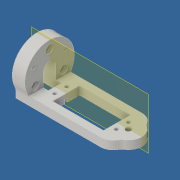
# Autodesk Inventor part: ServoMount
Saved by Autodesk Inventor 2016 SP1 (Build 200210100, 210)
## iProperties
Created: 2016-03-20
Part Number: ServoMount
Material: ABS-Kunststoff
Document SubType Name: Modeling
Designer: 4ndreas
Density: 1.06 g/cm^3
Appearance: Glatt - weiß
Mass: 21.5528 g
Surface Area: 97.0469 cm^2
Volume: 20.3328 cm^3
Author: 4ndreas
Autodesk Inventor part; units mm, degrees
ref_plane "YZ Plane" through (0, 0, 0) normal (1, 0, 0) x (0, 1, 0)
ref_plane "XZ Plane" through (0, 0, 0) normal (0, 1, 0) x (-1, 0, 0)
ref_plane "XY Plane" through (0, 0, 0) normal (0, 0, 1) x (1, 0, 0)
sketch "Skizze1" plane through (0, 0, 0) normal (0, 0, 1) x (1, 0, 0)
  line L0 (40, -18.5) -> (0, -18.5) projected
  line L1 (0, -18.5) -> (0, 0.5) projected
  line L2 (0, 0.5) -> (40, 0.5) projected
  line L3 (40, 0.5) -> (40, -18.5) projected
  circle A0 centre (-4.25, -4.25) radius 2.25 projected
  circle A1 centre (-4.25, -13.75) radius 2.25 projected
  arc A2 (-6, 0) -> (-7, -1) centre (-6, -1) ccw projected
  line L4 (-7, -1) -> (-7, -17) projected
  arc A3 (-7, -17) -> (-6, -18) centre (-6, -17) ccw projected
  line L5 (0, -18) -> (-6, -18) projected
  line L6 (0, 0) -> (0, -18) projected
  line L7 (0, 0) -> (-6, 0) projected
  arc A4 (46, -18) -> (47, -17) centre (46, -17) ccw projected
  line L8 (40, -18) -> (46, -18) projected
  line L9 (40, 0) -> (40, -18) projected
  line L10 (40, 0) -> (46, 0) projected
  arc A5 (47, -1) -> (46, 0) centre (46, -1) ccw projected
  line L11 (47, -1) -> (47, -17) projected
  circle A6 centre (44.25, -4.25) radius 2.25 projected
  circle A7 centre (44.25, -13.75) radius 2.25 projected
  line L12 (-13, 7.5) -> (53, 7.5)
  line L13 (53, 7.5) -> (53, -25.5)
  line L14 (53, -25.5) -> (-13, -25.5)
  line L15 (-13, -25.5) -> (-13, 7.5)
  line L16 (-13, 7.5) -> (53, -25.5) construction
  line L17 (53, 7.5) -> (-13, -25.5) construction
  arc A8 (38.105, -14.6823) -> (47.5399, -3.0302) centre (43, -9) ccw projected
  line L18 (43, -9) -> (-7, -9) construction
  point P0 (20, -9)
  point P1 (20, -9)
  dimension "d0" = 6
  dimension "d15" = 7
  dimension "d16" = 6
  constraints: 14 end point, 4 midpoint, 2 parallel, 1 coincident, 1 horizontal, 1 perpendicular, 1 point on line, 1 other
  measures "d0" distance between parallel lines of L11 L13
  measures "d15" distance between parallel lines of L0 L14
  measures "d16" distance between parallel lines of L15 L4
extrude "Extrusion1" add sketch "Skizze1" along normal blind 8 contours L3 A8 L11 A4 L8 | L5 A3 L4 A2 L7 L1 | L3 L10 A5 L11 A8 | L12 L13 L14 L15
sketch "Skizze2" plane through (0, 0, 8) normal (0, 0, 1) x (1, 0, 0)
  circle A0 centre (-4.25, -13.75) radius 2.25 construction
  circle A1 centre (-4.25, -4.25) radius 2.25 construction
  circle A2 centre (44.25, -13.75) radius 2.25 construction
  circle A3 centre (44.25, -4.25) radius 2.25 construction
  line L0 (0, 0.5) -> (40, 0.5) construction
  line L1 (40, 0.5) -> (40, -18.5) construction
  line L2 (40, -18.5) -> (0, -18.5) construction
  line L3 (0, -18.5) -> (0, 0.5) construction
  line L4 (53, 7.5) -> (-13, 7.5) construction
  line L5 (-13, 7.5) -> (-13, -25.5) construction
  line L6 (-13, -25.5) -> (53, -25.5) construction
  line L7 (53, -25.5) -> (53, 7.5) construction
  line L8 (-13, -9) -> (53, -9) construction
  point P0 (0, 0)
  point P1 (49, -9)
  point P2 (10, -9)
  dimension "d10" = 39
  dimension "d11" = 10
  constraints: 2 end point, 2 midpoint, 2 point on line
  measures "d10" distance of point (10, -9) point (49, -9)
  measures "d11" distance from line of point (10, -9) L3
hole "Bohrung1" at (49, -9, 8) direction (0, 0, -1) diameter 4 end through all
sketch "Skizze3" plane through (0, 0, 0) normal (0, 0, -1) x (-1, 0, 0)
  circle A0 centre (-49, -9) radius 2 projected
  circle A1 centre (4.25, -13.75) radius 2.25 projected
  circle A2 centre (4.25, -4.25) radius 2.25 projected
  circle A3 centre (-44.25, -13.75) radius 2.25 projected
  circle A4 centre (-44.25, -4.25) radius 2.25 projected
  line L0 (-40, 0.5) -> (0, 0.5) projected
  line L1 (0, 0.5) -> (0, -18.5) projected
  line L2 (0, -18.5) -> (-40, -18.5) projected
  line L3 (-40, -18.5) -> (-40, 0.5) projected
  line L4 (13, 7.5) -> (-53, 7.5) projected
  line L5 (-53, 7.5) -> (-53, -25.5) projected
  line L6 (-53, -25.5) -> (13, -25.5) projected
  line L7 (13, -25.5) -> (13, 7.5) projected
  arc A5 (-53, 0.7082) -> (-53, -18.7082) centre (-49, -9) ccw
  line L8 (-53, 7.5) -> (-53, -25.5) projected
  line L9 (-53, 0.7082) -> (-53, -18.7082)
  point P0 (0, 0)
  dimension "d12" = 10.5
  constraints: 3 point on circle, 3 point on line, 2 end point, 1 centre point, 1 coincident
  measures "d12" radius of A5
extrude "Extrusion2" add sketch "Skizze3" against normal up to surface (8 mm away) contours L5 A5
sketch "Skizze4" plane through (-13, -25.5, 0) normal (-1, 0, 0) x (0, 0, 1)
  line L0 (0, 0) -> (0, 33) projected
  line L1 (0, 0) -> (8, 0) projected
  line L2 (8, 33) -> (8, 0) projected
  line L3 (0, 33) -> (8, 33) projected
  line L4 (0, 16.5) -> (17, 16.5) construction
  arc A0 (6.6077, 0) -> (6.6077, 33) centre (17, 16.5) ccw
  circle A1 centre (17, 16.5) radius 19.5 construction
  point P0 (0, 25.5)
  dimension "d18" = 39
  dimension "d19" = 17
  constraints: 2 centre point, 2 coincident, 2 end point, 2 point on circle, 2 point on line, 1 concentric, 1 midpoint, 1 perpendicular
  measures "d18" diameter of A1
  measures "d19" distance of L4.start L4.end
extrude "Extrusion3" add sketch "Skizze4" along normal blind 10
sketch "Skizze5" plane through (-23, -25.5, 0) normal (-1, 0, 0) x (0, 0, 1)
  line L0 (0, 33) -> (0, 0) projected
  line L1 (0, 0) -> (6.6077, 0) projected
  arc A0 (6.6077, 0) -> (6.6077, 33) centre (17, 16.5) ccw projected
  line L2 (6.6077, 33) -> (0, 33) projected
  circle A1 centre (17, 16.5) radius 13 construction
  line L3 (17, 16.5) -> (30, 16.5) construction
  line L4 (17, 16.5) -> (10.5, 27.7583) construction
  line L5 (17, 16.5) -> (10.5, 5.2417) construction
  point P0 (0, 25.5)
  dimension "d22" = 26
  dimension "d23" = 120
  dimension "d24" = 120
  constraints: 6 end point, 3 point on circle, 1 centre point, 1 coincident, 1 horizontal
  measures "d22" diameter of A1
  measures "d23" angle of L3 L4
  measures "d24" angle of L3 L5
sketch "Skizze6" plane through (0, -18.5, 0) normal (1, 0, 0) x (0, 0, -1)
  point P0 (0, 18.5)
  point P1 (-10.5, 20.7583)
  point P2 (-10.5, -1.7583)
  point P3 (-30, 9.5)
hole "Bohrung2" at (0, -20.2583, 10.5) at (0, 2.2583, 10.5) at (0, -9, 30) direction (-1, 0, 0) diameter 3 end through all counterbore diameter 6.5 counterbore depth 16
sketch "Skizze7" plane through (0, 0, 0) normal (0, 0, -1) x (-1, 0, 0)
  circle A0 centre (-49, -9) radius 2 projected
  circle A1 centre (4.25, -13.75) radius 2.25 projected
  circle A2 centre (4.25, -4.25) radius 2.25 projected
  circle A3 centre (-44.25, -13.75) radius 2.25 projected
  circle A4 centre (-44.25, -4.25) radius 2.25 projected
  line L0 (-40, 0.5) -> (0, 0.5) projected
  line L1 (0, 0.5) -> (0, -18.5) projected
  line L2 (0, -18.5) -> (-40, -18.5) projected
  line L3 (-40, -18.5) -> (-40, 0.5) projected
  line L4 (23, 7.5) -> (-53, 7.5) projected
  line L5 (-53, 7.5) -> (-53, 0.7082) projected
  arc A5 (-53, 0.7082) -> (-53, -18.7082) centre (-49, -9) ccw projected
  line L6 (-53, -18.7082) -> (-53, -25.5) projected
  line L7 (-53, -25.5) -> (23, -25.5) projected
  line L8 (23, 7.5) -> (23, -25.5) projected
  circle A6 centre (4.25, -13.75) radius 1.25
  circle A7 centre (4.25, -4.25) radius 1.25
  circle A8 centre (-44.25, -4.25) radius 1.25
  circle A9 centre (-44.25, -13.75) radius 1.25
  point P0 (0, 0)
  dimension "d32" = 2.5
  constraints: 4 centre point, 4 coincident, 3 equal radius
  measures "d32" diameter of A6
extrude "Extrusion4" add sketch "Skizze7" against normal up to surface (8 mm away) contours A1 | A2 | A3 | A4
sketch "Skizze8" plane through (0, 0, 8) normal (0, 0, 1) x (1, 0, 0)
  circle A0 centre (44.25, -13.75) radius 1.25 projected
  circle A1 centre (44.25, -4.25) radius 1.25 projected
  circle A2 centre (49, -9) radius 2 projected
  line L0 (-13, 4.335) -> (0, 4.335) projected
  line L1 (0, 4.335) -> (0, 0.5) projected
  line L2 (0, 0.5) -> (40, 0.5) projected
  line L3 (40, 0.5) -> (40, -18.5) projected
  line L4 (40, -18.5) -> (0, -18.5) projected
  line L5 (0, -18.5) -> (0, -22.335) projected
  line L6 (0, -22.335) -> (-13, -22.335) projected
  line L7 (-13, -22.335) -> (-13, -25.5) projected
  line L8 (-13, -25.5) -> (53, -25.5) projected
  line L9 (53, -25.5) -> (53, -18.7082) projected
  arc A3 (53, -18.7082) -> (53, 0.7082) centre (49, -9) ccw projected
  line L10 (53, 0.7082) -> (53, 7.5) projected
  line L11 (53, 7.5) -> (-13, 7.5) projected
  line L12 (-13, 7.5) -> (-13, 4.335) projected
  circle A4 centre (49, -9) radius 11.5
  point P0 (0, 0)
  dimension "d69" = 1
  constraints: 1 centre point, 1 coincident
  measures "d69" radial gap between concentric circles of A4 A3
extrude "Extrusion5" cut sketch "Skizze8" against normal blind 1.5 contours A4 L9 A3 L10 | L10 A3 L9 A4 L3 | L3 A4
sketch "Skizze9" plane through (0, 0, 0) normal (0, 0, -1) x (-1, 0, 0)
  point P0 (0, 0)
fillet "Rundung1" radius 2 2 edges at (40, -1.8411, 7.25) (40, -16.1589, 7.25)
fillet "Rundung2" radius 10 2 edges at (-18, -25.5, 6.6077) (-18, 7.5, 6.6077)
sketch "Skizze10" plane through (0, 0, 0) normal (0, 0, -1) x (-1, 0, 0)
  circle A0 centre (-44.25, -13.75) radius 1.25 projected
  circle A1 centre (-44.25, -4.25) radius 1.25 projected
  circle A2 centre (4.25, -4.25) radius 1.25 projected
  circle A3 centre (4.25, -13.75) radius 1.25 projected
  circle A4 centre (-49, -9) radius 2 projected
  line L0 (-40, 0.5) -> (0, 0.5) projected
  line L1 (0, 0.5) -> (0, -18.5) projected
  line L2 (0, -18.5) -> (-40, -18.5) projected
  line L3 (-40, -18.5) -> (-40, 0.5) projected
  line L4 (23, 7.5) -> (-53, 7.5) projected
  line L5 (-53, 7.5) -> (-53, 0.7082) projected
  arc A5 (-53, 0.7082) -> (-53, -18.7082) centre (-49, -9) ccw projected
  line L6 (-53, -18.7082) -> (-53, -25.5) projected
  line L7 (-53, -25.5) -> (23, -25.5) projected
  line L8 (23, 7.5) -> (23, -25.5) projected
  line L9 (-44.9585, -9) -> (-46.9793, -12.5)
  line L10 (-46.9793, -12.5) -> (-51.0207, -12.5)
  line L11 (-51.0207, -12.5) -> (-53.0415, -9)
  line L12 (-53.0415, -9) -> (-51.0207, -5.5)
  line L13 (-51.0207, -5.5) -> (-46.9793, -5.5)
  line L14 (-46.9793, -5.5) -> (-44.9585, -9)
  point P0 (0, 0)
  dimension "d39" = 7
  constraints: 12 end point, 1 coincident, 1 parallel, 13 other
  measures "d39" distance between parallel lines of L10 L13
extrude "Extrusion6" cut sketch "Skizze10" against normal blind 3 contours A4 | L9 L10 L11 L12 L13 L14
sketch "Skizze11" plane through (0, 0, 3) normal (0, 0, -1) x (-1, 0, 0)
  circle A0 centre (-49, -9) radius 2 projected
  circle A1 centre (-49, -9) radius 2 projected
  point P0 (0, 0)
extrude "Extrusion7" add sketch "Skizze11" against normal blind 0.2
sketch "Skizze12" plane through (-13, -25.5, 0) normal (1, 0, 0) x (0, 0, -1)
  arc A0 (-8, 29.835) -> (-8, 25.6817) centre (-10.5, 27.7583) ccw projected
  line L0 (-8, 33) -> (-8, 29.835) projected
  line L1 (-4.0385, 33) -> (-8, 33) projected
  arc A1 (-8.4322, 34.0169) -> (-4.0385, 33) centre (-4.0385, 43) ccw projected
  arc A2 (-8.4322, 34.0169) -> (-8.4322, -1.0169) centre (-17, 16.5) ccw projected
  arc A3 (-4.0385, 0) -> (-8.4322, -1.0169) centre (-4.0385, -10) ccw projected
  line L2 (-4.0385, 0) -> (-8, 0) projected
  line L3 (-8, 3.165) -> (-8, 0) projected
  arc A4 (-8, 7.3183) -> (-8, 3.165) centre (-10.5, 5.2417) ccw projected
  line L4 (-8, 25.6817) -> (-8, 7.3183) projected
  circle A5 centre (-30, 16.5) radius 3.25 projected
  line L5 (-23.5, 4) -> (-23.5, 29)
  line L6 (-17, 16.5) -> (-30, 16.5) construction
  point P0 (0, 25.5)
  point P1 (-23.5, 16.5)
  dimension "d44" = 25
  constraints: 4 end point, 2 midpoint, 1 horizontal, 1 vertical
  measures "d44" distance of L5.start L5.end
hole "Bohrung3" at (-13, -21.5, 23.5) at (-13, 3.5, 23.5) direction (-1, 0, 0) diameter 3 end through all
sketch "Skizze13" plane through (-23, -25.5, 0) normal (-1, 0, 0) x (0, 0, 1)
  circle A0 centre (23.5, 4) radius 1.5 projected
  circle A1 centre (23.5, 29) radius 1.5 projected
  circle A2 centre (10.5, 27.7583) radius 1.5 projected
  circle A3 centre (10.5, 5.2417) radius 1.5 projected
  circle A4 centre (30, 16.5) radius 1.5 projected
  line L0 (0, 33) -> (0, 0) projected
  line L1 (0, 0) -> (4.0385, 0) projected
  arc A5 (8.4322, -1.0169) -> (4.0385, 0) centre (4.0385, -10) ccw projected
  arc A6 (8.4322, -1.0169) -> (8.4322, 34.0169) centre (17, 16.5) ccw projected
  arc A7 (4.0385, 33) -> (8.4322, 34.0169) centre (4.0385, 43) ccw projected
  line L2 (4.0385, 33) -> (0, 33) projected
  line L3 (26.6754, 29) -> (25.0877, 26.25)
  line L4 (25.0877, 26.25) -> (21.9123, 26.25)
  line L5 (21.9123, 26.25) -> (20.3246, 29)
  line L6 (20.3246, 29) -> (21.9123, 31.75)
  line L7 (21.9123, 31.75) -> (25.0877, 31.75)
  line L8 (25.0877, 31.75) -> (26.6754, 29)
  line L9 (26.6754, 4) -> (25.0877, 1.25)
  line L10 (25.0877, 1.25) -> (21.9123, 1.25)
  line L11 (21.9123, 1.25) -> (20.3246, 4)
  line L12 (20.3246, 4) -> (21.9123, 6.75)
  line L13 (21.9123, 6.75) -> (25.0877, 6.75)
  line L14 (25.0877, 6.75) -> (26.6754, 4)
  point P0 (0, 25.5)
  dimension "d52" = 5.5
  constraints: 24 end point, 3 parallel, 2 coincident, 26 other
  measures "d52" distance between parallel lines of L7 L4
extrude "Extrusion8" cut sketch "Skizze13" against normal blind 5 contours A0 | A1 | L3 L4 L5 L6 L7 L8 | L9 L10 L11 L12 L13 L14
sketch "Skizze14" plane through (-13, -25.5, 0) normal (1, 0, 0) x (0, 0, -1)
  circle A0 centre (-23.5, 4) radius 1.5 projected
  circle A1 centre (-23.5, 29) radius 1.5 projected
  arc A2 (-8, 29.835) -> (-8, 25.6817) centre (-10.5, 27.7583) ccw projected
  line L0 (-8, 33) -> (-8, 29.835) projected
  line L1 (-4.0385, 33) -> (-8, 33) projected
  arc A3 (-8.4322, 34.0169) -> (-4.0385, 33) centre (-4.0385, 43) ccw projected
  arc A4 (-8.4322, 34.0169) -> (-8.4322, -1.0169) centre (-17, 16.5) ccw projected
  arc A5 (-4.0385, 0) -> (-8.4322, -1.0169) centre (-4.0385, -10) ccw projected
  line L2 (-4.0385, 0) -> (-8, 0) projected
  line L3 (-8, 3.165) -> (-8, 0) projected
  arc A6 (-8, 7.3183) -> (-8, 3.165) centre (-10.5, 5.2417) ccw projected
  line L4 (-8, 25.6817) -> (-8, 7.3183) projected
  circle A7 centre (-30, 16.5) radius 3.25 projected
  point P0 (0, 25.5)
hole "Bohrung4" at (-13, -9, 17) direction (-1, 0, 0) diameter 10 end through all
sketch "Skizze15" plane through (0, 0, 8) normal (0, 0, 1) x (1, 0, 0)
  line L0 (-23, 7.5) -> (-23, -25.5) projected
  circle A0 centre (-4.25, -4.25) radius 1.25 projected
  circle A1 centre (-4.25, -13.75) radius 1.25 projected
  line L1 (0, 0.1817) -> (-13, 0.1817) projected
  line L2 (-13, 0.1817) -> (-13, -18.1817) projected
  line L3 (-13, -18.1817) -> (0, -18.1817) projected
  line L4 (0, -18.1817) -> (0, 0.1817) projected
  line L5 (-13, -14) -> (-9, -14)
  line L6 (-9, -14) -> (-9, -4)
  line L7 (-9, -4) -> (-13, -4)
  line L8 (-13, -4) -> (-13, -14)
  line L9 (0, -9) -> (-13, -9) construction
  point P0 (0, 0)
  dimension "d62" = 4
  dimension "d63" = 10
  constraints: 10 end point, 2 midpoint, 2 parallel, 1 horizontal, 1 perpendicular, 1 point on line, 1 other
  measures "d62" distance between parallel lines of L6 L2
  measures "d63" distance between parallel lines of L7 L5
extrude "Extrusion9" cut sketch "Skizze15" against normal through all contours L7 L6 L5 L2
fillet "Rundung3" radius 10 2 edges at (53, 7.5, 4) (53, -25.5, 4)
fillet "Rundung4" radius 10 2 edges at (53, 0.7082, 3.25) (53, -18.7082, 3.25)
fillet "Rundung5" radius 1 2 edges at (52.5922, 1.9246, 7.25) (52.5922, -19.9246, 7.25)
ref_plane "Arbeitsebene1" through (0, -9, 0) normal (0, -1, 0) x (1, 0, 0)
sketch "Skizze17" plane through (0, -9, 0) normal (0, -1, 0) x (1, 0, 0)
  line L0 (-9, 0) -> (-9, 8) projected
  line L1 (-9, 8) -> (0, 8) projected
  line L2 (0, 8) -> (0, 0) projected
  line L3 (0, 0) -> (-9, 0) projected
  line L4 (-23, 12) -> (-13, 12) projected
  line L5 (-13, 12) -> (-13, 0) projected
  line L6 (-13, 0) -> (-23, 0) projected
  line L7 (-23, 0) -> (-23, 12) projected
  line L8 (53.0415, 0) -> (53.0415, 3) projected
  line L9 (53.0415, 3) -> (44.9585, 3) projected
  line L10 (44.9585, 3) -> (44.9585, 0) projected
  line L11 (44.9585, 0) -> (40, 0) projected
  line L12 (40, 0) -> (40, 6.5) projected
  line L13 (40, 6.5) -> (47, 6.5) projected
  line L14 (47, 6.5) -> (47, 3.2) projected
  line L15 (47, 3.2) -> (51, 3.2) projected
  line L16 (51, 3.2) -> (51, 6.5) projected
  line L17 (51, 6.5) -> (59.5, 6.5) projected
  line L18 (59.5, 6.5) -> (59.5, 0) projected
  line L19 (59.5, 0) -> (53.0415, 0) projected
  line L20 (-16, 33.25) -> (-16, 31.5) projected
  line L21 (-16, 31.5) -> (-23, 31.5) projected
  line L22 (-23, 31.5) -> (-23, 36.5) projected
  line L23 (-23, 36.5) -> (-13, 36.5) projected
  line L24 (-13, 36.5) -> (-13, 33.25) projected
  line L25 (-13, 33.25) -> (-16, 33.25) projected
  line L26 (-16, 28.5) -> (-16, 26.75) projected
  line L27 (-16, 26.75) -> (-13, 26.75) projected
  line L28 (-13, 26.75) -> (-13, 22) projected
  line L29 (-13, 22) -> (-23, 22) projected
  line L30 (-23, 22) -> (-23, 28.5) projected
  line L31 (-23, 28.5) -> (-16, 28.5) projected
  line L32 (0, 3) -> (-7, 0)
  line L33 (40, 3) -> (47, 0)
  line L34 (47, 0) -> (40, 0)
  dimension "d70" = 3
  dimension "d71" = 7
  dimension "d73" = 7
  dimension "d80" = 3
  constraints: 6 end point, 5 point on line, 1 horizontal
  measures "d70" distance from line of L32.start L3
  measures "d71" distance from line of L32.end L2
  measures "d73" distance from line of L33.end L12
  measures "d80" distance from line of L33.start L11
extrude "Extrusion10" cut sketch "Skizze17" along normal mid plane 2 contours L32 L2 L3 | L33 L34 L10 | L10 L11 L12 L33
thicken "Verdickung1" operation cut thickness 1 both sides no extend neighbours no toward (0, -1, 0) faces at (13.3333, -18.5, 4.7556)
thicken "Verdickung2" operation cut thickness 1 both sides no extend neighbours no toward (0, 1, 0) faces at (13.3333, 0.5, 4.7556)
sketch "Skizze19" plane through (-23, -25.5, 0) normal (-1, 0, 0) x (0, 0, 1)
  circle A0 centre (17, 16.5) radius 5 projected
  line L0 (25.0877, 31.75) -> (26.6754, 29) projected
  line L1 (26.6754, 29) -> (25.0877, 26.25) projected
  line L2 (25.0877, 26.25) -> (21.9123, 26.25) projected
  line L3 (21.9123, 26.25) -> (20.3246, 29) projected
  line L4 (20.3246, 29) -> (21.9123, 31.75) projected
  line L5 (21.9123, 31.75) -> (25.0877, 31.75) projected
  line L6 (25.0877, 6.75) -> (26.6754, 4) projected
  line L7 (26.6754, 4) -> (25.0877, 1.25) projected
  line L8 (25.0877, 1.25) -> (21.9123, 1.25) projected
  line L9 (21.9123, 1.25) -> (20.3246, 4) projected
  line L10 (20.3246, 4) -> (21.9123, 6.75) projected
  line L11 (21.9123, 6.75) -> (25.0877, 6.75) projected
  circle A1 centre (10.5, 27.7583) radius 1.5 projected
  circle A2 centre (10.5, 5.2417) radius 1.5 projected
  circle A3 centre (30, 16.5) radius 1.5 projected
  line L12 (0, 33) -> (0, 0) projected
  line L13 (0, 0) -> (4.0385, 0) projected
  arc A4 (8.4322, -1.0169) -> (4.0385, 0) centre (4.0385, -10) ccw projected
  arc A5 (8.4322, -1.0169) -> (8.4322, 34.0169) centre (17, 16.5) ccw projected
  arc A6 (4.0385, 33) -> (8.4322, 34.0169) centre (4.0385, 43) ccw projected
  line L14 (4.0385, 33) -> (0, 33) projected
  line L15 (43.8, 16.5) -> (-7.3, 16.5) projected
  line L16 (17, 16.5) -> (-17, 16.5) construction
  line L17 (17, 21.5) -> (-17, 21.5)
  line L18 (-17, 11.5) -> (17, 11.5)
  arc A7 (17, 11.5) -> (17, 21.5) centre (17, 16.5) ccw
  arc A8 (-17, 21.5) -> (-17, 11.5) centre (-17, 16.5) ccw
  circle A9 centre (17, 16.5) radius 5 projected
  point P0 (0, 25.5)
  point P1 (0, 16.5)
  constraints: 8 end point, 5 tangent, 4 point on circle, 2 centre point, 2 midpoint, 1 parallel, 1 point on line
extrude "Extrusion11" cut sketch "Skizze19" against normal up to surface (14 mm away) contours A0 L15 L12 L17 | L18 L12 L15 A0 | L12 L18 A8 L17
sketch "Skizze20" plane through (0, 0, 6.5) normal (0, 0, 1) x (1, 0, 0)
  line L0 (40, -19.5) -> (0, -19.5) projected
  line L1 (0, -19.5) -> (0, -22.335) projected
  line L2 (0, -22.335) -> (-13, -22.335) projected
  line L3 (-13, -22.335) -> (-13, -25.5) projected
  line L4 (-13, -25.5) -> (43.5286, -25.5) projected
  arc A0 (43.5286, -25.5) -> (51.0485, -22.0918) centre (43.5286, -15.5) ccw projected
  arc A1 (51.0485, -22.0918) -> (50.1928, -20.438) centre (50.2965, -21.4326) ccw projected
  arc A2 (42.4023, -18.4192) -> (50.1928, -20.438) centre (49, -9) ccw projected
  arc A3 (42.4023, -18.4192) -> (40, -18.5) centre (41.2549, -20.0573) ccw projected
  line L5 (40, -18.5) -> (40, -19.5) projected
  line L6 (-9, -14) -> (-13, -14) projected
  line L7 (-13, -14) -> (-13, -18.1817) projected
  line L8 (-13, -18.1817) -> (0, -18.1817) projected
  line L9 (0, -18.1817) -> (0, 0.1817) projected
  line L10 (0, 0.1817) -> (-13, 0.1817) projected
  line L11 (-13, 0.1817) -> (-13, -4) projected
  line L12 (-13, -4) -> (-9, -4) projected
  line L13 (-9, -4) -> (-9, -14) projected
  circle A4 centre (-4.25, -4.25) radius 1.25 projected
  circle A5 centre (-4.25, -13.75) radius 1.25 projected
  line L14 (0, 1.5) -> (40, 1.5) projected
  line L15 (40, 1.5) -> (40, 0.5) projected
  arc A6 (40, 0.5) -> (42.4023, 0.4192) centre (41.2549, 2.0573) ccw projected
  arc A7 (50.1928, 2.438) -> (42.4023, 0.4192) centre (49, -9) ccw projected
  arc A8 (50.1928, 2.438) -> (51.0485, 4.0918) centre (50.2965, 3.4326) ccw projected
  arc A9 (51.0485, 4.0918) -> (43.5286, 7.5) centre (43.5286, -2.5) ccw projected
  line L16 (43.5286, 7.5) -> (-13, 7.5) projected
  line L17 (-13, 7.5) -> (-13, 4.335) projected
  line L18 (-13, 4.335) -> (0, 4.335) projected
  line L19 (0, 4.335) -> (0, 1.5) projected
  line L20 (-23, -14) -> (-9, -14) projected
  line L21 (-9, -14) -> (-9, -4) projected
  line L22 (-9, -4) -> (-23, -4) projected
  line L23 (-23, -4) -> (-23, 7.8077) projected
  line L24 (-23, 7.8077) -> (-13, 7.8077) projected
  line L25 (-13, 7.8077) -> (-13, 7.5) projected
  line L26 (-13, 7.5) -> (43.5286, 7.5) projected
  arc A10 (51.0485, 4.0918) -> (43.5286, 7.5) centre (43.5286, -2.5) ccw projected
  arc A11 (50.1928, 2.438) -> (51.0485, 4.0918) centre (50.2965, 3.4326) ccw projected
  arc A12 (50.1928, 2.438) -> (42.4023, 0.4192) centre (49, -9) ccw projected
  arc A13 (40, 0.5) -> (42.4023, 0.4192) centre (41.2549, 2.0573) ccw projected
  line L27 (40, -18.5) -> (40, 0.5) projected
  arc A14 (42.4023, -18.4192) -> (40, -18.5) centre (41.2549, -20.0573) ccw projected
  arc A15 (42.4023, -18.4192) -> (50.1928, -20.438) centre (49, -9) ccw projected
  arc A16 (51.0485, -22.0918) -> (50.1928, -20.438) centre (50.2965, -21.4326) ccw projected
  arc A17 (51.0485, -22.0918) -> (52.0733, -20.695) centre (43.5286, -15.5) ccw projected
  arc A18 (54.9507, -17.651) -> (52.0733, -20.695) centre (60.618, -25.89) ccw projected
  arc A19 (54.9507, -17.651) -> (54.9507, -0.349) centre (49, -9) ccw projected
  arc A20 (52.0733, 2.695) -> (54.9507, -0.349) centre (60.618, 7.89) ccw projected
  arc A21 (52.0733, 2.695) -> (51.0485, 4.0918) centre (43.5286, -2.5) ccw projected
  line L28 (-23, -25.8077) -> (-23, -14) projected
  line L29 (-13, -25.8077) -> (-23, -25.8077) projected
  line L30 (-13, -25.5) -> (-13, -25.8077) projected
  line L31 (43.5286, -25.5) -> (-13, -25.5) projected
  arc A22 (43.5286, -25.5) -> (51.0485, -22.0918) centre (43.5286, -15.5) ccw projected
  line L32 (40, 0.5) -> (40, 1.5) projected
  line L33 (40, 1.5) -> (0, 1.5) projected
  line L34 (0, 1.5) -> (0, -19.5) projected
  line L35 (0, -19.5) -> (40, -19.5) projected
  line L36 (40, -19.5) -> (40, -18.5) projected
  circle A23 centre (44.25, -13.75) radius 1.25 projected
  circle A24 centre (44.25, -4.25) radius 1.25 projected
  circle A25 centre (-4.25, -4.25) radius 1.25 projected
  circle A26 centre (-4.25, -13.75) radius 1.25 projected
  circle A27 centre (49, -9) radius 2 projected
  line L37 (-13, 0.1817) -> (-13, 4.335)
  line L38 (-13, -22.335) -> (-13, -18.1817)
  point P0 (0, 0)
  constraints: 4 end point, 1 collinear, 1 vertical
extrude "Extrusion12" cut sketch "Skizze20" along normal through all contours L5 A3 A2 A1 A0 L4 L3 L2 L1 L0 | L1 L2 L38 L8 L34 | L8 L7 L6 L13 L12 L11 L10 L9 | L15 L14 L19 L18 L17 L16 A9 A8 A7 A6 | L10 L37 L18 L19 L34
equation "\"d16\" = d0"
equation "\"d24\" = d23"
equation "\"d73\" = d71"
equation "\"d80\" = d70"
